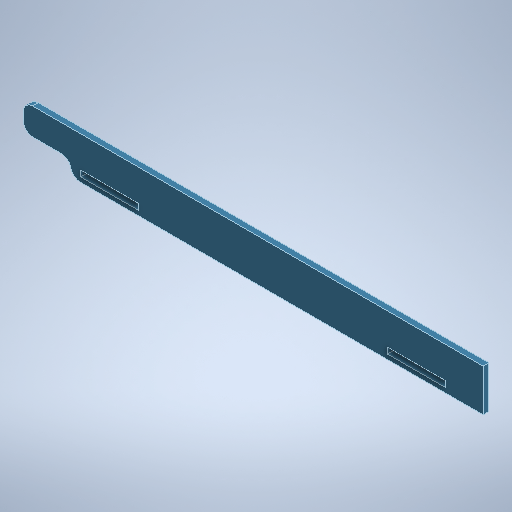
# Autodesk Inventor part: Starting Path Wall
Saved by Autodesk Inventor 2025.4 (Build 294407000, 407)
## iProperties
Created: 2026-05-20
Part Number: Starting Path Wall
Material: Generic
Document SubType Name: Sheet Metal
Designer: lenovo
Density: 1 g/cm^3
Sheet Metal Rule: Default_mm
Appearance: Default(1)
Author: lenovo
Autodesk Inventor part; units mm, degrees
ref_plane "YZ Plane" through (0, 0, 0) normal (1, 0, 0) x (0, 1, 0)
ref_plane "XZ Plane" through (0, 0, 0) normal (0, 1, 0) x (-1, 0, 0)
ref_plane "XY Plane" through (0, 0, 0) normal (0, 0, 1) x (1, 0, 0)
sketch "Sketch1" plane through (0, 0, 0) normal (0, 0, 1) x (1, 0, 0)
  line L0 (-120, -11) -> (120, -11)
  line L1 (120, -11) -> (120, 11)
  line L2 (120, 11) -> (-120, 11)
  line L3 (-120, 11) -> (-120, -11)
  line L4 (-120, -11) -> (120, 11) construction
  line L5 (120, -11) -> (-120, 11) construction
  line L6 (-90, -5.43) -> (-59.93, -5.43)
  line L7 (-59.93, -5.43) -> (-59.93, -8.5)
  line L8 (-59.93, -8.5) -> (-90, -8.5)
  line L9 (-90, -8.5) -> (-90, -5.43)
  line L10 (-90, -5.43) -> (-59.93, -8.5) construction
  line L11 (-59.93, -5.43) -> (-90, -8.5) construction
  line L12 (100.14, -5.42) -> (70.07, -5.42)
  line L13 (70.07, -5.42) -> (70.07, -8.5)
  line L14 (70.07, -8.5) -> (100.14, -8.5)
  line L15 (100.14, -8.5) -> (100.14, -5.42)
  line L16 (100.14, -5.42) -> (70.07, -8.5) construction
  line L17 (70.07, -5.42) -> (100.14, -8.5) construction
  line L18 (-120, -11) -> (-95, -11)
  line L19 (-95, -11) -> (-95, -3)
  line L20 (-95, -3) -> (-120, -3)
  line L21 (-120, -3) -> (-120, -11)
  point P0 (0, 0)
  point P1 (-74.965, -6.965)
  point P2 (85.105, -6.96)
  point P3 (-95, -11)
  dimension "d0" = 240
  dimension "d1" = 22
  dimension "d2" = 30.07
  dimension "d3" = 3.07
  dimension "d4" = 2.5
  dimension "d5" = 30
  dimension "d6" = 30.07
  dimension "d7" = 3.08
  dimension "d8" = 2.5
  dimension "d9" = 130
  dimension "d12" = 25
  dimension "d13" = 8
  measures "d0" distance of L2.end L1.end
  measures "d1" distance between parallel lines of L2 L0
  measures "d2" distance of L7.end L8.end
  measures "d3" distance of L6.end L7.end
  measures "d4" distance between parallel lines of L0 L8
  measures "d5" distance between parallel lines of L9 L3
  measures "d6" distance of L14.end L13.end
  measures "d7" distance of L13.end L12.end
  measures "d8" distance between parallel lines of L14 L0
  measures "d9" distance between parallel lines of L7 L13
  measures "d12" distance of L20.end L19.end
  measures "d13" distance of L19.end L18.end
extrude "Plate1" add sketch "Sketch1" along normal blind 3 contours L19 L20 L3 L2 L1 L0
fillet "Corner Round1" radius 5 4 edges at (-120, 11, 1.5) (-120, -3, 1.5) (-95, -3, 1.5) (-95, -11, 1.5)
equation "\"d10\" = Thickness"
equation "\"BendRadius\" = Thickness"
equation "\"BendReliefWidth\" = Thickness"
equation "\"BendReliefDepth\" = 0.5 * Thickness"
equation "\"CornerReliefSize\" = 4 * Thickness"
equation "\"MinimumRemnant\" = 2 * Thickness"
equation "\"TransitionRadius\" = BendRadius"
equation "\"JacobiRadiusSize\" = BendRadius"
equation "\"GapSize\" = Thickness"
equation "\"Thickness\" = 3"
body "Solid1"
